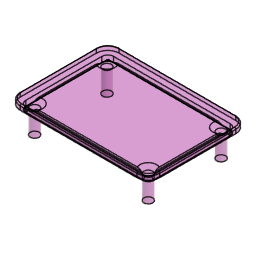
GlitchPixel404_A1_Top v1 (Autodesk Fusion 360 design; units mm, degrees)
Autodesk Fusion 360 part; units mm, degrees
note: some values were not read from the file. Chosen so that the rebuilt part matches the saved one: which pieces of a blend or face edit are solid.
sketch "Sketch1" plane through (0, 0, 0) normal (0, 0, 1) x (1, 0, 0)
  line L0 (3.6786, 4.5101) -> (49.6786, 4.5101) construction
  line L1 (51.6786, 6.5101) -> (51.6786, 36.5101) construction
  line L2 (49.6786, 38.5101) -> (3.6786, 38.5101) construction
  line L3 (1.6786, 36.5101) -> (1.6786, 6.5101) construction
  arc A0 (3.6786, 38.5101) -> (1.6786, 36.5101) centre (3.6786, 36.5101) ccw construction
  arc A1 (51.6786, 36.5101) -> (49.6786, 38.5101) centre (49.6786, 36.5101) ccw construction
  arc A2 (49.6786, 4.5101) -> (51.6786, 6.5101) centre (49.6786, 6.5101) ccw construction
  arc A3 (1.6786, 6.5101) -> (3.6786, 4.5101) centre (3.6786, 6.5101) ccw construction
  line L4 (3.6786, 2.0101) -> (49.6786, 2.0101)
  arc A4 (49.6786, 2.0101) -> (54.1786, 6.5101) centre (49.6786, 6.5101) ccw
  line L5 (54.1786, 6.5101) -> (54.1786, 36.5101)
  arc A5 (54.1786, 36.5101) -> (49.6786, 41.0101) centre (49.6786, 36.5101) ccw
  line L6 (49.6786, 41.0101) -> (3.6786, 41.0101)
  arc A6 (3.6786, 41.0101) -> (-0.8214, 36.5101) centre (3.6786, 36.5101) ccw
  line L7 (-0.8214, 36.5101) -> (-0.8214, 6.5101)
  arc A7 (-0.8214, 6.5101) -> (3.6786, 2.0101) centre (3.6786, 6.5101) ccw
  circle A8 centre (49.0786, 7.1101) radius 1.75
  circle A9 centre (49.0786, 35.8101) radius 1.75
  circle A10 centre (4.2786, 7.1101) radius 1.75
  circle A11 centre (4.4786, 35.4101) radius 1.75
  point P0 (1.6786, 38.5101)
  dimension "d3" = 2
  dimension "d4" = 2
  dimension "d5" = 2
  dimension "d6" = 2
  dimension "d7" = 50
  dimension "d8" = 34
  dimension "d9" = 2.5
  dimension "d15" = 3.5
  dimension "d16" = 2.6
  dimension "d17" = 2.6
  dimension "d18" = 3.5
  dimension "d19" = 28.7
  dimension "d20" = 2.6
  dimension "d21" = 3.5
  dimension "d22" = 44.8
  dimension "d23" = 2.6
  dimension "d24" = 3.5
  dimension "d25" = 44.6
  dimension "d26" = 28.3
  constraint horizontal L0
  constraint vertical L1
  constraint horizontal L2
  constraint vertical L3
  constraint coincident P0 L2
  constraint coincident P0 L3
  constraint tangent L2 A0
  constraint tangent L3 A0
  constraint tangent L1 A1
  constraint tangent L2 A1
  constraint tangent L0 A2
  constraint tangent L1 A2
  constraint tangent L0 A3
  constraint tangent L3 A3
  measures "d3" radius of A0
  measures "d4" radius of A1
  measures "d5" radius of A2
  measures "d6" radius of A3
  measures "d7" distance of L1 L3
  measures "d8" distance of L0 L2
  measures "d15" diameter of A8
  measures "d16" distance of L0 A8.centre
  measures "d17" distance of L1 A8.centre
  measures "d18" diameter of A9
  measures "d19" vertical distance of A8.centre A9.centre
  measures "d20" distance of L1 A9.centre
  measures "d21" diameter of A10
  measures "d22" horizontal distance of A8.centre A10.centre
  measures "d23" distance of L0 A10.centre
  measures "d24" diameter of A11
  measures "d25" horizontal distance of A9.centre A11.centre
  measures "d26" vertical distance of A10.centre A11.centre
extrude "Extrude1" add sketch "Sketch1" against normal blind 2 contours L4 A4 L5 A5 L6 A6 L7 A7 | A8 | A9 | A10 | A11
sketch "Sketch5" plane through (0, 0, -2) normal (0, 0, -1) x (-1, 0, 0)
  arc A0 (-3.6786, 2.0101) -> (0.8214, 6.5101) centre (-3.6786, 6.5101) ccw
  line L0 (-49.6786, 2.0101) -> (-3.6786, 2.0101)
  arc A1 (-54.1786, 6.5101) -> (-49.6786, 2.0101) centre (-49.6786, 6.5101) ccw
  line L1 (-54.1786, 36.5101) -> (-54.1786, 6.5101)
  arc A2 (-49.6786, 41.0101) -> (-54.1786, 36.5101) centre (-49.6786, 36.5101) ccw
  line L2 (-3.6786, 41.0101) -> (-49.6786, 41.0101)
  arc A3 (0.8214, 36.5101) -> (-3.6786, 41.0101) centre (-3.6786, 36.5101) ccw
  line L3 (0.8214, 6.5101) -> (0.8214, 36.5101)
  line L4 (-51.9786, 36.5101) -> (-51.9786, 6.5101)
  arc A4 (-51.9786, 6.5101) -> (-49.6785, 4.2101) centre (-49.6786, 6.5101) ccw
  line L5 (-49.6785, 4.2101) -> (-3.6786, 4.2101)
  arc A5 (-3.6786, 4.2101) -> (-1.3786, 6.5101) centre (-3.6786, 6.5101) ccw
  line L6 (-1.3786, 6.5101) -> (-1.3786, 36.5101)
  arc A6 (-1.3786, 36.5101) -> (-3.6786, 38.8101) centre (-3.6786, 36.5101) ccw
  line L7 (-3.6786, 38.8101) -> (-49.6786, 38.8101)
  arc A7 (-49.6786, 38.8101) -> (-51.9786, 36.5101) centre (-49.6786, 36.5101) ccw
  line L8 (-50.4786, 36.5101) -> (-50.4786, 6.5101)
  arc A8 (-50.4786, 6.5101) -> (-49.6786, 5.7101) centre (-49.6786, 6.5101) ccw
  line L9 (-49.6786, 5.7101) -> (-3.6786, 5.7101)
  arc A9 (-3.6786, 5.7101) -> (-2.8786, 6.5101) centre (-3.6786, 6.5101) ccw
  line L10 (-2.8786, 6.5101) -> (-2.8786, 36.5101)
  arc A10 (-2.8786, 36.5101) -> (-3.6786, 37.3101) centre (-3.6786, 36.5101) ccw
  line L11 (-3.6786, 37.3101) -> (-49.6786, 37.3101)
  arc A11 (-49.6786, 37.3101) -> (-50.4786, 36.5101) centre (-49.6786, 36.5101) ccw
  dimension "d47" = 2.2
  dimension "d48" = 3.7
extrude "Extrude7" add sketch "Sketch5" along normal blind 2 contours L4 A4 L5 A5 L6 A6 L7 A7
chamfer "Chamfer1" distance 1.3 angle 45 8 edges at (26.6786, 37.3101, -4) (3.1129, 37.0758, -4) (2.8786, 21.5101, -4) (3.1129, 5.9444, -4) (26.6786, 5.7101, -4) (50.2442, 5.9444, -4) (50.4786, 21.5101, -4) (50.2442, 37.0758, -4)
extrude "Extrude8" add sketch "Sketch1" against normal blind 10.6 from surface at -2 contours A8 | A9 | A10 | A11
fillet "Fillet1" radius 0.5 8 edges at (54.1786, 21.5101, 0) (52.8606, 39.6921, 0) (26.6786, 41.0101, 0) (0.4966, 39.6921, 0) (-0.8214, 21.5101, 0) (0.4966, 3.3281, 0) (26.6786, 2.0101, 0) (52.8605, 3.3281, 0)
fillet "Fillet2" radius 1.5 4 edges at (5.516, 8.3475, -2) (47.8411, 8.3475, -2) (6.2286, 35.4101, -2) (47.7794, 34.6376, -2)
equation "d15 = d24"
equation "d18 = d24"
equation "d21 = d24"
equation "d48 = d47 + 1.5 mm"
named bodies: "GlitchPixel404_A1_Base"
